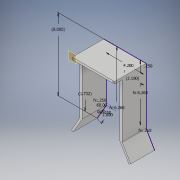
# Autodesk Inventor part: U-Part Gen 2
Saved by Autodesk Inventor 2019 (Build 230136000, 136)
## iProperties
Created: 2019-10-05
Part Number: U-Part Gen 2
Material: Generic
Document SubType Name: Modeling
Designer: Delta
Density: 1 g/cm^3
Appearance: Default
Author: Delta
Autodesk Inventor part; units mm, degrees
ref_plane "YZ Plane" through (0, 0, 0) normal (1, 0, 0) x (0, 1, 0)
ref_plane "XZ Plane" through (0, 0, 0) normal (0, 1, 0) x (-1, 0, 0)
ref_plane "XY Plane" through (0, 0, 0) normal (0, 0, 1) x (1, 0, 0)
sketch "Sketch1" plane through (0, 0, 0) normal (0, 0, 1) x (1, 0, 0)
  line L0 (0, 0) -> (119.38, 0)
  line L1 (119.38, 0) -> (119.38, -6.35)
  line L2 (119.38, -6.35) -> (0, -6.35)
  line L3 (0, -6.35) -> (0, 0)
  line L4 (119.38, 0) -> (113.03, 0)
  line L5 (113.03, 0) -> (113.03, -159.2059)
  line L6 (113.03, -159.2059) -> (119.38, -159.2059)
  line L7 (119.38, -159.2059) -> (119.38, 0)
  line L8 (0, 0) -> (6.35, 0)
  line L9 (6.35, 0) -> (6.35, -159.2059)
  line L10 (6.35, -159.2059) -> (0, -159.2059)
  line L11 (0, -159.2059) -> (0, 0)
  line L12 (0, -152.8559) -> (25.4, -152.8559) construction
  line L13 (6.35, -159.2059) -> (38.1, -159.2059) construction
  line L14 (0, -159.2059) -> (-23.8125, -200.4504)
  line L15 (6.35, -159.2059) -> (-19.05, -203.2)
  line L16 (-23.8125, -200.4504) -> (-19.05, -203.2)
  line L17 (59.69, 0) -> (59.69, -59.745)
  line L18 (119.38, -159.2059) -> (143.1925, -200.4504)
  line L19 (113.03, -159.2059) -> (138.43, -203.2)
  line L20 (143.1925, -200.4504) -> (138.43, -203.2)
  dimension "d1" = 6.35
  dimension "d2" = 6.35
  dimension "d3" = 159.2059
  dimension "d5" = 159.2059
  dimension "d6" = 6.35
  dimension "d13" = 6.35
  dimension "d15" = 106.68
  dimension "d28" = 0
  dimension "d29" = 60
  dimension "d30" = 50.8
  dimension "d31" = 53.34
  dimension "d32" = 203.2
  dimension "d33" = 43.9941
  constraints: 42 end point, 6 parallel, 5 horizontal, 4 perpendicular, 2 symmetric about line, 1 midpoint, 1 point on line, 1 vertical
  measures "d1" distance of L0.end L1.end
  measures "d2" distance of L6.end L5.end
  measures "d3" distance of L5.end L4.end
  measures "d5" distance between parallel lines of L10 L0
  measures "d6" distance of L12.start L10.end
  measures "d13" distance between parallel lines of L11 L9
  measures "d15" distance between parallel lines of L5 L9
  measures "d28" angle of L14 L15
  measures "d29" angle of L10 L15
  measures "d30" distance from line of L9.end L16
  measures "d31" distance between parallel lines of L5 L17
  measures "d32" distance from line of L0 L15.end
  measures "d33" distance from line of L10 L15.end
ref_plane "Work Plane2" through (0, 0, 88.9) normal (0, 0, 1) x (1, 0, 0)
sketch "Sketch3" plane through (0, 0, 88.9) normal (0, 0, 1) x (1, 0, 0)
  line L0 (0, 0) -> (0, -159.2059) projected
  line L1 (6.35, -159.2059) -> (6.35, -6.35) projected
  line L2 (119.38, 0) -> (0, 0) projected
  line L3 (119.38, -159.2059) -> (119.38, 0) projected
  circle A0 centre (3.175, -3.175) radius 1.778
  circle A1 centre (116.205, -3.175) radius 1.778
  line L4 (119.38, -6.35) -> (0, -6.35) projected
  dimension "d18" = 3.175
  dimension "d19" = 6.35
  dimension "d20" = 3.175
  dimension "d21" = 3.175
  dimension "d22" = 3.175
  dimension "d23" = 3.556
  dimension "d24" = 3.556
  dimension "d38" = 119.38
  dimension "d39" = 6.35
  constraints: 2 centre point, 2 coincident, 1 other
  measures "d18" distance from line of L0 point (3.175, -3.175)
  measures "d19" distance between parallel lines of L0 L1
  measures "d20" distance from line of L2 point (3.175, -3.175)
  measures "d21" distance from line of L2 point (116.205, -3.175)
  measures "d22" distance from line of L3 point (116.205, -3.175)
  measures "d23" diameter of A0
  measures "d24" diameter of A1
  measures "d38" distance of L2.start L0.start
extrude "Extrusion4" add sketch "Sketch1" along normal blind 88.9 contours L0 L9 L2 L3 | L0 L17 L2 L9 | L0 L5 L2 L17 | L0 L1 L2 L5
extrude "Extrusion5" add sketch "Sketch1" along normal blind 67.31 contours L0 L9 L2 L3 | L2 L9 L10 L11 | L10 L15 L16 L14 | L0 L1 L2 L5 | L2 L7 L6 L5 | L6 L18 L20 L19
extrude "Extrusion6" cut sketch "Sketch3" against normal through all contours A0 | A1
equation "\"d2\" = d1"
equation "\"d3\" = d5"
equation "\"d6\" = d4"
equation "\"d13\" = d2"
equation "\"d18\" = 0.5 * d19"
equation "\"d20\" = 0.5 * d39"
equation "\"d21\" = d20"
equation "\"d22\" = d18"
equation "\"d4\" = d2"
body "Solid2"
